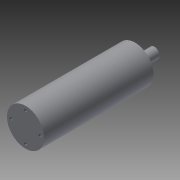
# Autodesk Inventor part: Part80
Saved by Autodesk Inventor 2015 (Build 190159000, 159)
## iProperties
Created: 2015-01-12
Part Number: Part80
Material: Generic
Document SubType Name: Modeling
Designer: mastkee16
Density: 1 g/cm^3
Appearance: Default
Author: mastkee16
Autodesk Inventor part; units mm, degrees
ref_plane "YZ Plane" through (0, 0, 0) normal (1, 0, 0) x (0, 1, 0)
ref_plane "XZ Plane" through (0, 0, 0) normal (0, 1, 0) x (-1, 0, 0)
ref_plane "XY Plane" through (0, 0, 0) normal (0, 0, 1) x (1, 0, 0)
sketch "Sketch1" plane through (0, 0, 0) normal (0, 0, 1) x (1, 0, 0)
  circle A0 centre (0, 0) radius 22.4676
  circle A1 centre (0, 0) radius 6.35
  point P0 (0, 17.5006)
  point P1 (-17.5006, 0)
  point P2 (0, -17.5006)
  point P3 (17.5006, 0)
  dimension "d0" = 44.9351
  dimension "d1" = 12.7
  dimension "d6" = 35.0012
  dimension "d7" = 17.5006
  dimension "d8" = 17.5006
  dimension "d9" = 17.5006
  dimension "d10" = 17.5006
  constraints: 2 centre point, 2 coincident
  measures "d0" diameter of A0
  measures "d1" diameter of A1
  measures "d6" distance of point (0, -17.501) point (0, 17.501)
  measures "d7" distance of point (0, 17.501) point (0, 0)
  measures "d8" distance of point (-17.501, 0) point (0, 0)
  measures "d9" distance of point (17.501, 0) point (0, 0)
  measures "d10" distance of point (0, 0) point (0, -17.501)
extrude "Extrusion1" add sketch "Sketch1" along normal blind 132.715 contours A0 | A1
extrude "Extrusion2" add sketch "Sketch1" against normal blind 23.5128 contours A1
hole "Hole1" at (0, 17.5006, 0) at (-17.5006, 0, 0) at (0, -17.5006, 0) at (17.5006, 0, 0) direction (0, 0, 1) diameter 3.5052 end through all
thread "Thread1" size "6-32 UNC" class "2B" standard "ANSI Unified Screw Threads" full length
thread "Thread2" size "6-32 UNC" class "2B" standard "ANSI Unified Screw Threads" full length
thread "Thread3" size "6-32 UNC" class "2B" standard "ANSI Unified Screw Threads" full length
thread "Thread4" size "6-32 UNC" class "2B" standard "ANSI Unified Screw Threads" full length
body "Solid1"
